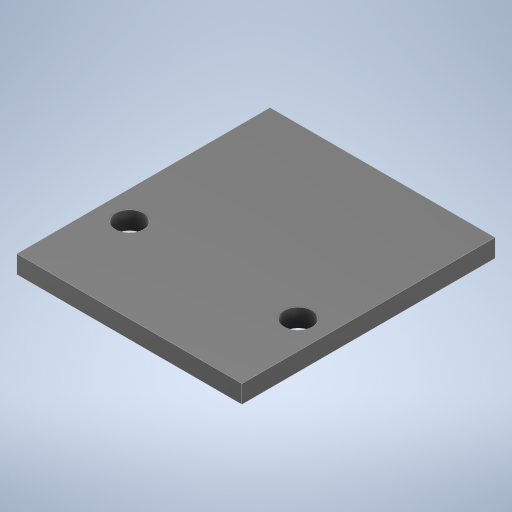
# Autodesk Inventor part: SUSTAINA-SCI-TO-HDMI-BOARD
Saved by Autodesk Inventor 2024.2 (Build 282272000, 272)
## iProperties
Created: 2024-02-11
Part Number: SUSTAINA-SCI-TO-HDMI-BOARD
Material: CFRP
Document SubType Name: Modeling
Designer: Masato Kubotera
Appearance: Smooth - Black
Surface Area: 10.415 cm^2
Volume: 0.704292 cm^3
Author: Masato Kubotera
Autodesk Inventor part; units mm, degrees
ref_plane "YZ Plane" through (0, 0, 0) normal (1, 0, 0) x (0, 1, 0)
ref_plane "XZ Plane" through (0, 0, 0) normal (0, 1, 0) x (-1, 0, 0)
ref_plane "XY Plane" through (0, 0, 0) normal (0, 0, 1) x (1, 0, 0)
sketch "Sketch1" plane through (0, 0, 0) normal (0, 0, 1) x (1, 0, 0)
  line L0 (11.25, 10) -> (-11.25, 10)
  line L1 (-11.25, 10) -> (-11.25, -10)
  line L2 (-11.25, -10) -> (11.25, -10)
  line L3 (11.25, -10) -> (11.25, 10)
  line L4 (11.25, 10) -> (-11.25, -10) construction
  line L5 (-11.25, 10) -> (11.25, -10) construction
  line L6 (0, 10) -> (0, -10) construction
  line L7 (11.25, 0) -> (-11.25, 0) construction
  line L8 (0, -10) -> (0, 10) construction
  line L9 (3.75, -7.5) -> (3.75, 7.5) construction
  point P0 (0, 0)
  point P1 (3.75, 0)
  dimension "d0" = 22.5
  dimension "d1" = 20
  dimension "d18" = 7.5
  dimension "d19" = 15
  constraints: 20 end point, 7 midpoint, 2 parallel, 2 symmetric about line, 1 horizontal, 1 perpendicular, 1 point on line, 1 vertical
  measures "d0" distance of L2.end L1.end
  measures "d1" distance of L1.end L0.end
  measures "d18" distance between parallel lines of L3 L9
  measures "d19" distance of L9.start L9.end
extrude "Extrusion1" add sketch "Sketch1" along normal blind 1.6
hole "Hole1" at (3.75, -7.5, 0) at (3.75, 7.5, 0) direction (0, 0, 1) diameter 2.5 end through all
body "Solid1"
